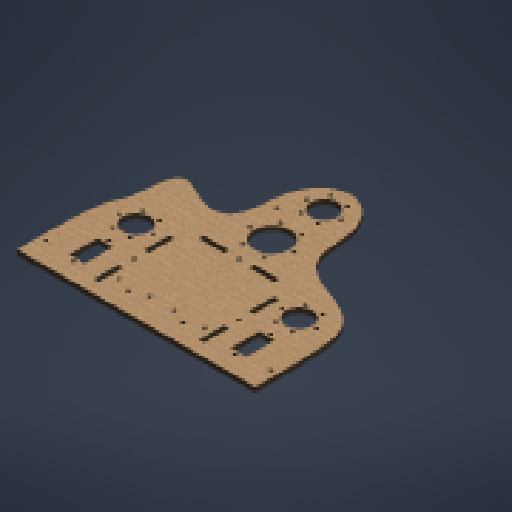
# Autodesk Inventor part: Cart_Floor
Saved by Autodesk Inventor 2024.1 (Build 281209000, 209)
## iProperties
Created: 2023-08-03
Part Number: Cart_Floor
Material: MDF Medium Density Fiberboard
Document SubType Name: Modeling
Designer: jaege
Density: 0.8 g/cm^3
Appearance: Cardboard - Corrugated
Author: jaege
Autodesk Inventor part; units mm, degrees
ref_plane "YZ Plane" through (0, 0, 0) normal (1, 0, 0) x (0, 1, 0)
ref_plane "XZ Plane" through (0, 0, 0) normal (0, 1, 0) x (-1, 0, 0)
ref_plane "XY Plane" through (0, 0, 0) normal (0, 0, 1) x (1, 0, 0)
sketch "Sketch1" plane through (0, 0, 0) normal (0, 1, 0) x (-1, 0, 0)
  line L0 (-40, -40) -> (40, -40) construction
  line L1 (40, -40) -> (40, 40) construction
  line L2 (40, 40) -> (-40, 40) construction
  line L3 (-40, 40) -> (-40, -40) construction
  line L4 (-40, 40) -> (40, 40) construction
  line L5 (40, 40) -> (40, 59.5) construction
  line L6 (40, 59.5) -> (-40, 59.5) construction
  line L7 (-40, 59.5) -> (-40, 40) construction
  circle A0 centre (-65, -24.9396) radius 10.5
  circle A1 centre (0, -68.5) radius 14
  line L8 (-44, 40) -> (44, 40) construction
  line L9 (44, 40) -> (44, -44) construction
  line L10 (44, -44) -> (-44, -44) construction
  line L11 (-44, -44) -> (-44, 40) construction
  line L12 (-100, 59.5) -> (100, 59.5) construction
  line L13 (100, 59.5) -> (100, -140.5) construction
  line L14 (100, -140.5) -> (-100, -140.5) construction
  line L15 (-100, -140.5) -> (-100, 59.5) construction
  line L16 (0, -180.5) -> (0, 99.5) construction
  circle A2 centre (-51.25, -24.9396) radius 1.5
  circle A3 centre (-65, -24.9396) radius 17 construction
  line L17 (-54.5, -24.9396) -> (-48, -24.9396) construction
  circle A4 centre (-58.125, -13.0317) radius 1.5
  circle A5 centre (-71.875, -13.0317) radius 1.5
  circle A6 centre (-78.75, -24.9396) radius 1.5
  circle A7 centre (-71.875, -36.8474) radius 1.5
  circle A8 centre (-58.125, -36.8474) radius 1.5
  circle A9 centre (0, -110) radius 10.5
  circle A10 centre (13.75, -110) radius 1.5
  circle A11 centre (0, -110) radius 17 construction
  line L18 (10.5, -110) -> (17, -110) construction
  circle A12 centre (6.875, -98.0922) radius 1.5
  circle A13 centre (-6.875, -98.0922) radius 1.5
  circle A14 centre (-13.75, -110) radius 1.5
  circle A15 centre (-6.875, -121.9078) radius 1.5
  circle A16 centre (6.875, -121.9078) radius 1.5
  line L19 (-70.6, 27.5) -> (-58.4, 27.5) construction
  line L20 (-58.4, 27.5) -> (-58.4, -4.7) construction
  line L21 (-58.4, -4.7) -> (-70.6, -4.7) construction
  line L22 (-70.6, -4.7) -> (-70.6, 27.5) construction
  circle A17 centre (-64.5, 25.5) radius 1.5
  circle A18 centre (-64.5, -2.7) radius 1.5
  line L23 (-64.5, 27.5) -> (-64.5, -4.7) construction
  line L24 (-70.6, 11.4) -> (-58.4, 11.4) construction
  circle A19 centre (-64.5, 16.5) radius 2.5 construction
  circle A20 centre (17.25, -68.5) radius 1.5
  circle A21 centre (0, -68.5) radius 20.5 construction
  line L25 (14, -68.5) -> (20.5, -68.5) construction
  circle A22 centre (8.625, -53.5611) radius 1.5
  circle A23 centre (-8.625, -53.5611) radius 1.5
  circle A24 centre (-17.25, -68.5) radius 1.5
  circle A25 centre (-8.625, -83.4389) radius 1.5
  circle A26 centre (8.625, -83.4389) radius 1.5
  line L26 (0, 40) -> (-95, 40) construction
  line L27 (-95, 40) -> (-95, 14.5) construction
  line L28 (-95, 14.5) -> (0, 14.5) construction
  line L29 (0, 14.5) -> (0, 40) construction
  line L30 (0, 40) -> (-95, 40) construction
  line L31 (-95, 40) -> (-95, 55.5) construction
  line L32 (-95, 55.5) -> (0, 55.5) construction
  line L33 (0, 55.5) -> (0, 40) construction
  circle A27 centre (-64.5, 16.5) radius 17.5 construction
  line L34 (-44, 14.5) -> (-85, 14.5) construction
  line L35 (-85, 14.5) -> (-85, 55.5) construction
  line L36 (-85, 55.5) -> (-44, 55.5) construction
  line L37 (-44, 55.5) -> (-44, 14.5) construction
  line L38 (-82, 16.5) -> (-82, -24.9396) construction
  circle A28 centre (65, -24.9396) radius 10.5
  circle A29 centre (51.25, -24.9396) radius 1.5
  circle A30 centre (65, -24.9396) radius 17 construction
  line L39 (54.5, -24.9396) -> (48, -24.9396) construction
  circle A31 centre (58.125, -13.0317) radius 1.5
  circle A32 centre (71.875, -13.0317) radius 1.5
  circle A33 centre (78.75, -24.9396) radius 1.5
  circle A34 centre (71.875, -36.8474) radius 1.5
  circle A35 centre (58.125, -36.8474) radius 1.5
  line L40 (70.6, 27.5) -> (58.4, 27.5) construction
  line L41 (58.4, 27.5) -> (58.4, -4.7) construction
  line L42 (58.4, -4.7) -> (70.6, -4.7) construction
  line L43 (70.6, -4.7) -> (70.6, 27.5) construction
  circle A36 centre (64.5, 25.5) radius 1.5
  circle A37 centre (64.5, -2.7) radius 1.5
  line L44 (64.5, 27.5) -> (64.5, -4.7) construction
  line L45 (70.6, 11.4) -> (58.4, 11.4) construction
  circle A38 centre (64.5, 16.5) radius 2.5 construction
  line L46 (0, 40) -> (95, 40) construction
  line L47 (95, 40) -> (95, 14.5) construction
  line L48 (95, 14.5) -> (0, 14.5) construction
  line L49 (0, 40) -> (95, 40) construction
  line L50 (95, 40) -> (95, 55.5) construction
  line L51 (95, 55.5) -> (0, 55.5) construction
  circle A39 centre (64.5, 16.5) radius 17.5 construction
  line L52 (44, 14.5) -> (85, 14.5) construction
  line L53 (85, 14.5) -> (85, 55.5) construction
  line L54 (85, 55.5) -> (44, 55.5) construction
  line L55 (82, 16.5) -> (82, -24.9396) construction
  line L56 (95, 40) -> (-95, 40)
  line L57 (95, 40) -> (95, 14.5)
  line L58 (-95, 40) -> (-95, 14.5)
  spline S0 degree 4 poles (-95, 14.5) (-95, 2.9745) (-92.5859, -15.0646) (-100.8312, -52.3699) (-16.3507, -57.8128) (-37.7982, -109.7894) (0, -145.5519) (37.7982, -109.7894) (16.3507, -57.8128) (100.8312, -52.3699) (92.5859, -15.0646) (95, 2.9745) (95, 14.5) knots 0 0 0 0 0 0.141322 0.242902 0.345989 0.449799 0.550201 0.654011 0.757098 0.858678 1 1 1 1 1
  line L59 (-65, -24.9396) -> (-65, -41.9396) construction
  line L60 (-95, 14.5) -> (-82.6777, -42.6172) construction
  line L61 (-30, -40) -> (-10, -40)
  line L62 (-10, -40) -> (-10, -44)
  line L63 (-10, -44) -> (-30, -44)
  line L64 (-30, -44) -> (-30, -40)
  line L65 (-44, -30) -> (-40, -30)
  line L66 (-40, -30) -> (-40, -10)
  line L67 (-40, -10) -> (-44, -10)
  line L68 (-44, -10) -> (-44, -30)
  line L69 (-44, 30) -> (-40, 30)
  line L70 (-40, 30) -> (-40, 10)
  line L71 (-40, 10) -> (-44, 10)
  line L72 (-44, 10) -> (-44, 30)
  line L73 (30, -40) -> (10, -40)
  line L74 (10, -40) -> (10, -44)
  line L75 (10, -44) -> (30, -44)
  line L76 (30, -44) -> (30, -40)
  line L77 (44, -30) -> (40, -30)
  line L78 (40, -30) -> (40, -10)
  line L79 (40, -10) -> (44, -10)
  line L80 (44, -10) -> (44, -30)
  line L81 (44, 30) -> (40, 30)
  line L82 (40, 30) -> (40, 10)
  line L83 (40, 10) -> (44, 10)
  line L84 (44, 10) -> (44, 30)
  line L85 (-70.6, 22.65) -> (-58.4, 22.65)
  line L86 (-58.4, 22.65) -> (-58.4, 0.15)
  line L87 (-58.4, 0.15) -> (-70.6, 0.15)
  line L88 (-70.6, 0.15) -> (-70.6, 22.65)
  line L89 (70.6, 22.65) -> (58.4, 22.65)
  line L90 (58.4, 22.65) -> (58.4, 0.15)
  line L91 (58.4, 0.15) -> (70.6, 0.15)
  line L92 (70.6, 0.15) -> (70.6, 22.65)
  circle A40 centre (22, 24.5) radius 1.55 construction
  circle A41 centre (10, 19.5) radius 1.55 construction
  circle A42 centre (34, 19.5) radius 1.55 construction
  circle A43 centre (90, 22) radius 1.55 construction
  circle A44 centre (10, 19.5) radius 1.5
  circle A45 centre (22, 24.5) radius 1.5
  circle A46 centre (34, 19.5) radius 1.5
  circle A47 centre (90, 22) radius 1.5
  circle A48 centre (-22, 24.5) radius 1.55 construction
  circle A49 centre (-10, 19.5) radius 1.55 construction
  circle A50 centre (-34, 19.5) radius 1.55 construction
  circle A51 centre (-90, 22) radius 1.55 construction
  circle A52 centre (-10, 19.5) radius 1.5
  circle A53 centre (-22, 24.5) radius 1.5
  circle A54 centre (-34, 19.5) radius 1.5
  circle A55 centre (-90, 22) radius 1.5
  point P0 (0, 0)
  point P1 (0, 59.5)
  point P2 (0, -40)
  point P3 (40, 0)
  point P4 (0, -44)
  point P5 (0, -140.5)
  point P6 (-64.5, 11.4)
  point P7 (-95, 47.75)
  point P8 (-47, 16.5)
  point P9 (-82, 16.5)
  point P10 (0, -48)
  point P11 (0, -89)
  point P12 (0, -93)
  point P13 (64.5, 11.4)
  point P14 (95, 47.75)
  point P15 (47, 16.5)
  point P16 (82, 16.5)
  point P17 (-35, -68.5)
  point P18 (-25, -110)
  point P19 (0, -131)
  point P20 (25, -110)
  point P21 (35, -68.5)
  point P22 (82.6777, -42.6172)
  point P23 (-93.8388, -14.0586)
  point P24 (93.8388, -14.0586)
  point P25 (-88.8388, -14.0586)
  point P26 (-17, -110)
  point P27 (0, -127)
  point P28 (0, -40)
  point P29 (-42, 30)
  point P30 (-58.4, 11.4)
  dimension "d5" = 21
  dimension "d6" = 28
  dimension "d19" = 21
  dimension "d2" = 80
  dimension "d4" = 80
  dimension "d7" = 4
  dimension "d8" = 4
  dimension "d9" = 200
  dimension "d10" = 200
  dimension "d11" = 3
  dimension "d12" = 34
  dimension "d15" = 360
  dimension "d20" = 3
  dimension "d21" = 34
  dimension "d22" = 360
  dimension "d23" = 32.2
  dimension "d24" = 12.2
  dimension "d25" = 3
  dimension "d26" = 5
  dimension "d27" = 9
  dimension "d28" = 28.2
  dimension "d29" = 3
  dimension "d30" = 6.5
  dimension "d33" = 360
  dimension "d36" = 25.5
  dimension "d37" = 41
  dimension "d39" = 95
  dimension "d40" = 35
  dimension "d42" = 4
  dimension "d44" = 39
  dimension "d45" = 3
  dimension "d46" = 21
  dimension "d47" = 3
  dimension "d48" = 3
  dimension "d49" = 4
  dimension "d50" = 4
  dimension "d51" = 25
  dimension "d52" = 45
  dimension "d53" = 5
  dimension "d54" = 35
  dimension "d55" = 8
  dimension "d56" = 4
  dimension "d57" = 20
  dimension "d58" = 20
  dimension "d60" = 10
  dimension "d61" = 10
  dimension "d62" = 20
  dimension "d64" = 10
  dimension "d65" = 22.5
  dimension "d66" = 3
  constraints: 184 end point, 82 horizontal alignment, 48 centre point, 24 parallel, 23 equal radius, 22 coincident, 18 midpoint, 18 point on circle, 15 horizontal, 12 perpendicular, 12 point on line, 8 vertical alignment, 4 vertical, 3 collinear, 2 tangent, 1 symmetric about line, 67 other
  measures "d2" distance of L6.end L5.end
  measures "d4" distance of L0.end L1.end
  measures "d7" distance between parallel lines of L11 L3
  measures "d8" distance between parallel lines of L10 L0
  measures "d9" distance of L12.start L12.end
  measures "d10" distance of L14.end L12.start
  measures "d11" diameter of A2
  measures "d12" diameter of A3
  measures "d20" diameter of A10
  measures "d21" diameter of A11
  measures "d23" distance of L21.end L19.start
  measures "d24" distance of L19.start L19.end
  measures "d25" diameter of A17
  measures "d26" diameter of A19
  measures "d27" distance of A19.centre A17.centre
  measures "d28" distance of A18.centre A17.centre
  measures "d29" diameter of A20
  measures "d36" distance of L26.end L27.end
  measures "d37" distance between parallel lines of L32 L28
  measures "d39" distance of L27.end L28.end
  measures "d40" diameter of A27
  measures "d42" vertical distance of L12.start L31.end
  measures "d44" distance from line of A27.centre L32
  measures "d45" distance from line of L11 A27.start
  measures "d46" distance of L21.end L59.start
  measures "d47" distance from line of A27.end L35
  measures "d48" distance from line of L37 A27.start
  measures "d49" distance of A21.end point (0, -44)
  measures "d50" distance of A11.end point (0, -89)
  measures "d51" distance of L59.start L60.end
  measures "d53" distance of point (-88.839, -14.059) point (-93.839, -14.059)
  measures "d54" distance of point (0, -68.5) point (-35, -68.5)
  measures "d55" distance of point (-17, -110) point (-25, -110)
  measures "d56" distance of point (0, -131) point (0, -127)
  measures "d57" distance of L66.end L65.end
  measures "d58" distance of L69.end L70.end
  measures "d60" distance from line of L0.start L65
  measures "d61" distance of L61.start L0.start
  measures "d62" distance of L61.start L61.end
  measures "d64" distance from line of L26 point (-42, 30)
  measures "d65" distance of L85.end L86.end
  measures "d66" diameter of A44
extrude "Extrusion1" add sketch "Sketch1" along normal blind 4
sketch "Sketch3" plane through (0, 4, 0) normal (0, 1, 0) x (1, 0, 0)
  line L0 (-17.9772, 90.6455) -> (-17.9772, 93.6455) construction
  line L1 (-17.9772, 93.6455) -> (-21.9772, 93.6455) construction
  line L2 (-21.9772, 90.6455) -> (-21.9772, 93.6455) construction
  line L3 (-17.9772, 90.6455) -> (-21.9772, 90.6455) construction
  line L4 (-17.9772, 90.6455) -> (-21.9772, 93.6455) construction
  circle A0 centre (-19.9772, 92.1455) radius 1.5
  point P0 (0, 0)
  dimension "d69" = 3
  constraints: 2 end point, 1 centre point, 1 midpoint
  measures "d69" diameter of A0
extrude "Extrusion3" cut sketch "Sketch3" against normal up to next
sketch "Sketch4" plane through (0, 4, 0) normal (0, 1, 0) x (1, 0, 0)
  spline S0 degree 4 poles (95, -14.5) (95, -2.9745) (92.5859, 15.0646) (100.8312, 52.3699) (16.3507, 57.8128) (37.7982, 109.7894) (0, 145.5519) (-37.7982, 109.7894) (-16.3507, 57.8128) (-100.8312, 52.3699) (-92.5859, 15.0646) (-95, -2.9745) (-95, -14.5) knots 0 0 0 0 0 0.141322 0.242902 0.345989 0.449799 0.550201 0.654011 0.757098 0.858678 1 1 1 1 1 projected
  spline S1 degree 4 poles (-32.4176, 72.2818) (-34.5106, 68.831) (-40.3469, 63.961) (-55.1943, 65.4418) (-73.2386, 79.1276) (-88.6181, 77.807) (-83.4801, 44.4126) (-88.6623, 35.5) knots 0.13656 0.13656 0.13656 0.13656 0.13656 0.303115 0.458634 0.634836 1 1 1 1 1 projected
  point P0 (0, 0)
  constraints: 1 other
extrude "Extrusion4" add sketch "Sketch4" against normal up to surface (4 mm away)
sketch "Sketch5" plane through (0, 4, 0) normal (0, 1, 0) x (1, 0, 0)
  circle A0 centre (-19.9772, 92.1455) radius 1.5 construction
  line L0 (95, -40) -> (95, -14.5) construction
  line L1 (-95, -14.5) -> (-95, -40) construction
  line L2 (-95, -40) -> (95, -40) construction
  circle A1 centre (90, -22) radius 1.5 construction
  circle A2 centre (34, -19.5) radius 1.5 construction
  circle A3 centre (10, -19.5) radius 1.5 construction
  circle A4 centre (-90, -22) radius 1.5 construction
  circle A5 centre (-34, -19.5) radius 1.5 construction
  circle A6 centre (-22, -24.5) radius 1.5 construction
  circle A7 centre (-10, -19.5) radius 1.5 construction
  circle A8 centre (-64.5, -25.5) radius 1.5 construction
  circle A9 centre (64.5, -25.5) radius 1.5 construction
  circle A10 centre (22, -24.5) radius 1.5 construction
  line L3 (-70.6, -0.15) -> (-58.4, -0.15) construction
  line L4 (-58.4, -0.15) -> (-58.4, -22.65) construction
  line L5 (-58.4, -22.65) -> (-70.6, -22.65) construction
  line L6 (-70.6, -22.65) -> (-70.6, -0.15) construction
  line L7 (70.6, -22.65) -> (58.4, -22.65) construction
  line L8 (58.4, -22.65) -> (58.4, -0.15) construction
  line L9 (58.4, -0.15) -> (70.6, -0.15) construction
  line L10 (70.6, -0.15) -> (70.6, -22.65) construction
  line L11 (-40, -30) -> (-44, -30) construction
  line L12 (-44, -30) -> (-44, -10) construction
  line L13 (-44, -10) -> (-40, -10) construction
  line L14 (-40, -10) -> (-40, -30) construction
  line L15 (-40, 30) -> (-40, 10) construction
  line L16 (-40, 10) -> (-44, 10) construction
  line L17 (-44, 10) -> (-44, 30) construction
  line L18 (-44, 30) -> (-40, 30) construction
  line L19 (-10, 40) -> (-30, 40) construction
  line L20 (-30, 40) -> (-30, 44) construction
  line L21 (-30, 44) -> (-10, 44) construction
  line L22 (-10, 44) -> (-10, 40) construction
  line L23 (44, -30) -> (40, -30) construction
  line L24 (40, -30) -> (40, -10) construction
  line L25 (40, -10) -> (44, -10) construction
  line L26 (44, -10) -> (44, -30) construction
  line L27 (44, 30) -> (44, 10) construction
  line L28 (44, 10) -> (40, 10) construction
  line L29 (40, 10) -> (40, 30) construction
  line L30 (40, 30) -> (44, 30) construction
  line L31 (30, 40) -> (10, 40) construction
  line L32 (10, 40) -> (10, 44) construction
  line L33 (10, 44) -> (30, 44) construction
  line L34 (30, 44) -> (30, 40) construction
  circle A11 centre (-78.75, 24.9396) radius 1.5 construction
  circle A12 centre (-64.5, 2.7) radius 1.5 construction
  circle A13 centre (-58.125, 36.8474) radius 1.5 construction
  circle A14 centre (-71.875, 36.8474) radius 1.5 construction
  circle A15 centre (-71.875, 13.0317) radius 1.5 construction
  circle A16 centre (-58.125, 13.0317) radius 1.5 construction
  circle A17 centre (-51.25, 24.9396) radius 1.5 construction
  circle A18 centre (-65, 24.9396) radius 10.5 construction
  circle A19 centre (-8.625, 83.4389) radius 1.5 construction
  circle A20 centre (8.625, 83.4389) radius 1.5 construction
  circle A21 centre (17.25, 68.5) radius 1.5 construction
  circle A22 centre (8.625, 53.5611) radius 1.5 construction
  circle A23 centre (-8.625, 53.5611) radius 1.5 construction
  circle A24 centre (-17.25, 68.5) radius 1.5 construction
  circle A25 centre (64.5, 2.7) radius 1.5 construction
  circle A26 centre (6.875, 98.0922) radius 1.5 construction
  circle A27 centre (13.75, 110) radius 1.5 construction
  circle A28 centre (0, 110) radius 10.5 construction
  circle A29 centre (-6.875, 121.9078) radius 1.5 construction
  circle A30 centre (6.875, 121.9078) radius 1.5 construction
  circle A31 centre (-6.875, 98.0922) radius 1.5 construction
  circle A32 centre (-13.75, 110) radius 1.5 construction
  circle A33 centre (58.125, 36.8474) radius 1.5 construction
  circle A34 centre (71.875, 36.8474) radius 1.5 construction
  circle A35 centre (78.75, 24.9396) radius 1.5 construction
  circle A36 centre (71.875, 13.0317) radius 1.5 construction
  circle A37 centre (58.125, 13.0317) radius 1.5 construction
  circle A38 centre (51.25, 24.9396) radius 1.5 construction
  circle A39 centre (0, 68.5) radius 14 construction
  circle A40 centre (65, 24.9396) radius 10.5 construction
  line L35 (-10, 44) -> (10, 40) construction
  line L36 (-44, 10) -> (-40, -10) construction
  line L37 (40, -10) -> (44, 10) construction
  circle A41 centre (-42, 0) radius 1.5
  circle A42 centre (0, 42) radius 1.5
  circle A43 centre (42, 0) radius 1.5
  point P0 (0, 0)
  dimension "d74" = 3
  constraints: 6 end point, 3 centre point, 3 midpoint, 2 equal radius, 1 perpendicular, 3 other
  measures "d74" diameter of A41
extrude "Extrusion5" cut sketch "Sketch5" against normal up to next
body "Solid1"
